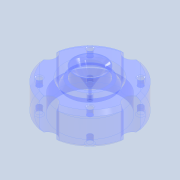
# Autodesk Inventor part: cpd_1.9_p3_v11
Saved by Autodesk Inventor 2021 (Build 250183000, 183)
## iProperties
Created: 2021-12-08
Part Number: cpd_1.9_p3_v11
Material: Generic
Document SubType Name: Modeling
Designer: tomos
Density: 1 g/cm^3
Appearance: Clear - Blue
Author: tomos
Autodesk Inventor part; units mm, degrees
ref_plane "YZ Plane" through (0, 0, 0) normal (1, 0, 0) x (0, 1, 0)
ref_plane "XZ Plane" through (0, 0, 0) normal (0, 1, 0) x (-1, 0, 0)
ref_plane "XY Plane" through (0, 0, 0) normal (0, 0, 1) x (1, 0, 0)
sketch "Sketch1" plane through (0, 0, 0) normal (0, 0, 1) x (1, 0, 0)
  line L0 (0, 0) -> (0, 22.2922) construction
  line L1 (0, 0) -> (22.0718, 0) construction
  line L2 (0.35, 3.25) -> (0.35, 6.6208)
  line L3 (0.35, 6.6208) -> (3.6, 12.25)
  line L4 (3.6, 12.25) -> (4.6, 12.25)
  line L5 (4.6, 12.25) -> (4.6, 9.25)
  line L6 (4.6, 9.25) -> (5.5, 9.25)
  line L7 (5.5, 9.25) -> (6.5, 7.5179)
  line L8 (6.5, 7.5179) -> (7.5, 9.25)
  line L9 (7.5, 9.25) -> (12.5, 9.25)
  line L10 (12.5, 9.25) -> (12.5, 0)
  line L11 (9.075, 5.25) -> (0.7, 5.25)
  line L12 (0.7, 3.25) -> (0.35, 3.25)
  line L13 (9.075, 0) -> (12.5, 0)
  line L14 (0.7, 5.25) -> (0.7, 3.25)
  line L15 (9.075, 0) -> (9.075, 5.25)
  dimension "d0" = 12.5
  dimension "d4" = 0.35
  dimension "d5" = 2
  dimension "d7" = 30
  dimension "d8" = 3
  dimension "d9" = 4.6
  dimension "d10" = 1
  dimension "d14" = 6.5
  dimension "d15" = 60
  dimension "d16" = 2
  dimension "d51" = 0.7
  dimension "d54" = 4
  dimension "d55" = 5.25
  dimension "d56" = 9.075
  constraints: 32 end point, 5 vertical, 3 perpendicular, 3 point on line, 2 horizontal, 1 parallel
  measures "d0" distance between parallel lines of L10 L0
  measures "d4" distance between parallel lines of L2 L0
  measures "d5" distance between parallel lines of L12 L11
  measures "d7" angle of L3 L0
  measures "d8" distance of L4.end L5.end
  measures "d9" distance between parallel lines of L5 L0
  measures "d10" distance of L3.end L4.end
  measures "d14" distance from line of L7.end L0
  measures "d15" angle of L8 L7
  measures "d16" distance of L8.end L6.end
  measures "d51" distance between parallel lines of L0 L14
  measures "d54" distance between parallel lines of L11 L9
  measures "d55" distance between parallel lines of L1 L11
  measures "d56" distance between parallel lines of L15 L0
revolve "Revolution1" add sketch "Sketch1" angle 360 about axis through (0, 0, 0) along (0, 1, 0)
chamfer "Chamfer1" distance 0.75 angle 45 1 edges at (-3.6, 12.25, 0)
chamfer "Chamfer2" distance 1 angle 45 2 edges at (-12.5, 9.25, 0) (-12.5, 0, 0)
sketch "Sketch2" plane through (0, 0, 0) normal (0, -1, 0) x (1, 0, 0)
  circle A0 centre (0, 0) radius 10.5 construction
  line L0 (0, 0) -> (-14.6436, 0) construction
  line L1 (0, 0) -> (-11.2932, 11.2932) construction
  circle A1 centre (0, 0) radius 12.5
  circle A2 centre (-12.5, 0) radius 2.5
  circle A3 centre (-7.4246, 7.4246) radius 0.8
  point P0 (-12.25, 2.4875)
  point P1 (-12.25, -2.4875)
  dimension "d26" = 21
  dimension "d28" = 25
  dimension "d25" = 45
  dimension "d27" = 5
  dimension "d29" = 1.6
  constraints: 4 end point, 2 centre point, 2 coincident, 2 point on line, 1 horizontal, 6 other
  measures "d25" angle of L0 L1
  measures "d27" diameter of A2
  measures "d29" diameter of A3
extrude "Extrusion1" cut sketch "Sketch2" against normal blind 2 contours A3
extrude "Extrusion2" cut sketch "Sketch2" against normal through all contours A2 A1 picked at (-11.6481, 0)
chamfer "Chamfer3" distance 0.35 angle 45 1 edges at (-8.2246, 0, 7.4246)
pattern_circular "Circular Pattern1" count 4 over 360 about axis through (0, -10, 0) along (0, 1, 0) of "Extrusion2", "Extrusion1", "Chamfer3"
sketch "Sketch3" plane through (-12.5, 9.25, 0) normal (0, 1, 0) x (1, 0, 0)
  circle A0 centre (12.5, 0) radius 0.35 construction
  circle A1 centre (12.5, 0) radius 10.5 construction
  line L0 (12.5, 0) -> (30.51, 0) construction
  line L1 (12.5, 0) -> (26.5897, -14.0897) construction
  circle A2 centre (19.9246, -7.4246) radius 0.8
  dimension "d41" = 21
  dimension "d40" = 45
  dimension "d42" = 1.6
  constraints: 4 end point, 2 coincident, 1 centre point, 1 horizontal, 2 other
  measures "d40" angle of L1 L0
  measures "d42" diameter of A2
extrude "Extrusion3" cut sketch "Sketch3" against normal blind 2
chamfer "Chamfer4" distance 0.25 angle 45 1 edges at (6.6246, 9.25, 7.4246)
pattern_circular "Circular Pattern2" count 4 over 360 about axis through (0, -10, 0) along (0, 1, 0) of "Extrusion3", "Chamfer4"
chamfer "Chamfer5" distance 0.25 angle 45 1 edges at (-0.7, 3.25, 0)
equation "\"cutpipette_length\" = 5.25"
body "Solid1"
